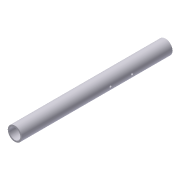
# Autodesk Inventor part: FE-00026
Saved by Autodesk Inventor 2012 (Build 160160000, 160)
## iProperties
Company: FIRST
Created: 2008-05-25
Part Number: FE-00026
Document SubType Name: Modeling
Designer: dfoster
Density: 1 g/cm^3
Description: Connecting Pin
Mass: 118.521 g
Surface Area: 672.502 cm^2
Volume: 118.521 cm^3
Material: Default
Title: Connecting Pin
Author: dfoster
Autodesk Inventor part; units mm, degrees
ref_plane "XZ Plane" through (0, 0, 0) normal (0, 1, 0) x (-1, 0, 0)
ref_plane "XY Plane" through (0, 0, 0) normal (0, 0, 1) x (1, 0, 0)
sketch "Sketch1" plane through (0, 0, 0) normal (0, 0, 1) x (1, 0, 0)
  circle A0 centre (0, 0) radius 13.0969
  circle A1 centre (0, 0) radius 16.6688
  dimension "d0" = 26.1938
  dimension "d1" = 33.3375
  constraints: 2 centre point, 1 coincident
  measures "d0" diameter of A0
  measures "d1" diameter of A1
extrude "Extrusion1" add sketch "Sketch1" along normal blind 355.6
ref_plane "Work Plane1" through (0, 0, 0) normal (1, 0, 0) x (0, 0, 1)
sketch "Sketch2" plane through (0, 0, 0) normal (1, 0, 0) x (0, 0, 1)
  circle A0 centre (146.05, 0) radius 2.4257
  line L0 (-71.12, 0) -> (426.72, 0) projected
  line L1 (355.6, 13.0969) -> (355.6, -13.0969) projected
  dimension "d5" = 4.8514
  dimension "d6" = 209.55
  constraints: 1 centre point, 1 point on line
  measures "d5" diameter of A0
  measures "d6" distance from line of A0.centre L1
extrude "Extrusion2" cut sketch "Sketch2" against normal mid plane 381
pattern_linear "Rectangular Pattern1" count 2 spacing 50.8 along (0, 0, -1) of "Extrusion2"
body "Solid1"
